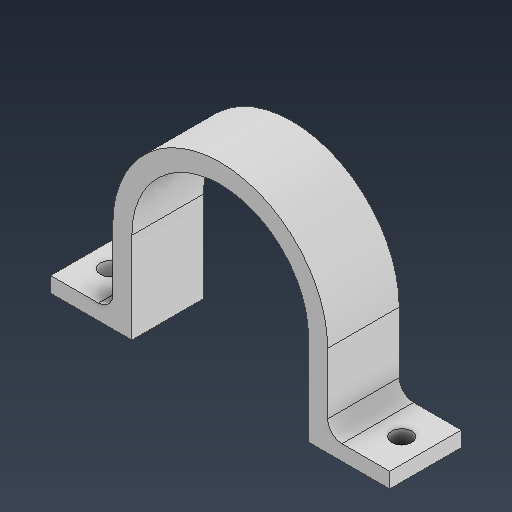
# Autodesk Inventor part: доп крепл мотора 25-26
Saved by Autodesk Inventor 2025 (Build 290162000, 162)
## iProperties
Created: 2025-09-24
Part Number: доп крепл мотора 25-26
Material: Типовые
Document SubType Name: Modeling
Designer: GameHD
Density: 1 g/cm^3
Appearance: По умолчанию
Author: GameHD
Autodesk Inventor part; units mm, degrees
ref_plane "YZ Plane" through (0, 0, 0) normal (1, 0, 0) x (0, 1, 0)
ref_plane "XZ Plane" through (0, 0, 0) normal (0, 1, 0) x (-1, 0, 0)
ref_plane "XY Plane" through (0, 0, 0) normal (0, 0, 1) x (1, 0, 0)
sketch "Эскиз1" plane through (0, 0, 0) normal (0, 0, 1) x (1, 0, 0)
  arc A0 (18.5, 0) -> (-18.5, 0) centre (0, 0) ccw
  line L0 (-22.5, 0) -> (22.5, 0)
  arc A1 (22.5, 0) -> (-22.5, 0) centre (0, 0) ccw
  line L1 (-22.5, 0) -> (-22.5, -12.8)
  line L2 (-22.5, -19) -> (-35.5, -19)
  line L3 (-35.5, -19) -> (-35.5, -15.8)
  line L4 (-35.5, -15.8) -> (-25.5, -15.8)
  arc A2 (-25.5, -15.8) -> (-22.5, -12.8) centre (-25.5, -12.8) ccw
  line L5 (-18.5, 0) -> (-18.5, -19)
  line L6 (-18.5, -19) -> (-22.5, -19)
  line L7 (0, 0) -> (0, 6.7823)
  line L8 (22.5, 0) -> (22.5, -12.8)
  line L9 (22.5, -19) -> (35.5, -19)
  line L10 (35.5, -19) -> (35.5, -15.8)
  line L11 (35.5, -15.8) -> (25.5, -15.8)
  arc A3 (22.5, -12.8) -> (25.5, -15.8) centre (25.5, -12.8) ccw
  line L12 (18.5, 0) -> (18.5, -19)
  line L13 (18.5, -19) -> (22.5, -19)
  dimension "d0" = 37
  dimension "d1" = 45
  dimension "d2" = 13
  dimension "d3" = 3.2
  dimension "d4" = 3
  constraints: 28 end point, 8 point on circle, 8 symmetric about line, 4 centre point, 4 perpendicular, 3 point on line, 3 tangent, 2 coincident, 2 horizontal, 2 vertical, 1 other
  measures "d0" diameter of A0
  measures "d1" diameter of A1
  measures "d2" distance of L2.start L2.end
  measures "d3" distance of L2.end L3.end
  measures "d4" radius of A2
extrude "Выдавливание1" add sketch "Эскиз1" along normal blind 15 contours A0 L0 A1 | L0 L8 A3 L11 L10 L9 L13 L12 | L5 L6 L2 L3 L4 A2 L1 L0
sketch "Эскиз2" plane through (-35.5, -15.8, 0) normal (0, 1, 0) x (1, 0, 0)
  line L0 (71, 0) -> (61, 0) projected
  line L1 (61, 0) -> (61, -15) projected
  line L2 (71, -15) -> (61, -15) projected
  line L3 (71, 0) -> (71, -15) projected
  line L4 (71, -7.5) -> (0, -7.5)
  line L5 (0, 0) -> (0, -15) projected
  line L6 (10, 0) -> (0, 0) projected
  line L7 (10, 0) -> (10, -15) projected
  line L8 (10, -15) -> (0, -15) projected
  line L9 (5, -15) -> (5, 0)
  circle A0 centre (5, -7.5) radius 2.1
  line L10 (35.5, 0) -> (35.5, -25.4)
  circle A1 centre (66, -7.5) radius 2.1
  dimension "d7" = 4.2
  constraints: 6 end point, 5 midpoint, 2 centre point, 1 symmetric about line, 1 vertical, 1 other
  measures "d7" diameter of A0
extrude "Выдавливание2" cut sketch "Эскиз2" against normal blind 20 contours A1 L4 | L4 A1 | A0 L9 L4 | L4 L9 A0 | L9 A0 L4 | L4 A0 L9
